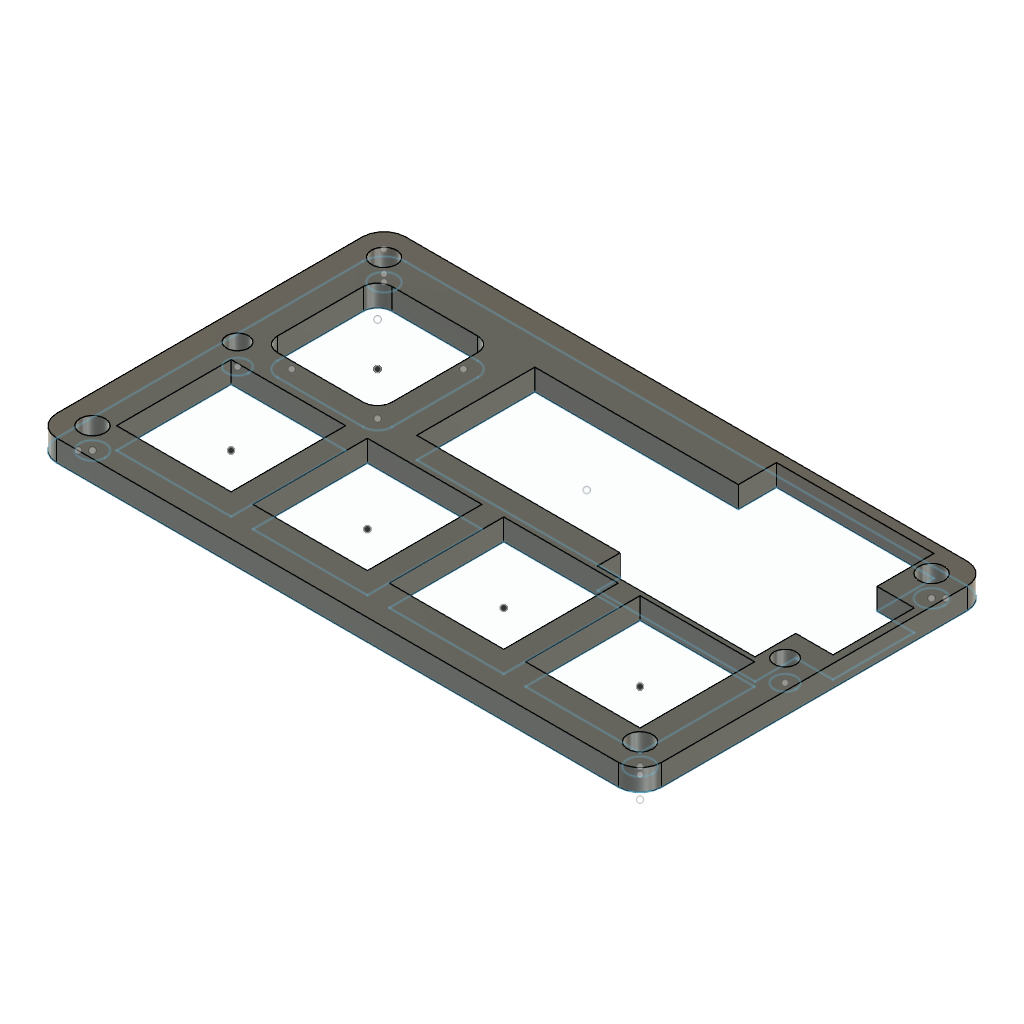
Hayai Upper midplate (Autodesk Fusion 360 design; units mm, degrees)
part number: 2026-09-20-16-56-58-125
Autodesk Fusion 360 part; units mm, degrees
sketch "Sketch1" plane through (0, 0, 0) normal (0, 0, 1) x (1, 0, 0)
  circle A0 centre (-38.26, 20.3675) radius 1.75
  circle A1 centre (38.26, 20.3675) radius 1.75
  circle A2 centre (38.26, -20.3675) radius 1.75
  circle A3 centre (-38.26, -20.3675) radius 1.75
  line L0 (14, 22.9575) -> (36, 22.9575)
  line L1 (36, 15) -> (36, 22.9575)
  line L2 (36, 15) -> (41.21, 15)
  line L3 (41.21, 15) -> (41.21, 3.65)
  line L4 (41.21, 3.65) -> (36, 3.65)
  line L5 (36, -2.0425) -> (36, 3.65)
  line L6 (36, -2.0425) -> (14, -2.0425)
  line L7 (-14.435, 1.1275) -> (-14.435, 17.6275)
  line L8 (-14.435, 1.1275) -> (14, 1.1275)
  line L9 (-14.435, 17.6275) -> (14, 17.6275)
  line L10 (14, -2.0425) -> (14, 1.1275)
  line L11 (14, 17.6275) -> (14, 22.9575)
  circle A4 centre (-38.26, -0.0995) radius 1.525
  circle A5 centre (38.26, -0.0995) radius 1.525
  line L12 (-39.26, 24.3675) -> (39.26, 24.3675)
  line L13 (42.26, 21.3675) -> (42.26, -21.3675)
  line L14 (39.26, -24.3675) -> (-39.26, -24.3675)
  line L15 (-42.26, -21.3675) -> (-42.26, 21.3675)
  arc A6 (-39.26, 24.3675) -> (-42.26, 21.3675) centre (-39.26, 21.3675) ccw
  arc A7 (42.26, 21.3675) -> (39.26, 24.3675) centre (39.26, 21.3675) ccw
  arc A8 (39.26, -24.3675) -> (42.26, -21.3675) centre (39.26, -21.3675) ccw
  arc A9 (-42.26, -21.3675) -> (-39.26, -24.3675) centre (-39.26, -21.3675) ccw
  line L16 (-22.19, 1.4035) -> (-34.19, 1.4035)
  line L17 (-36.19, 3.4035) -> (-36.19, 15.4035)
  line L18 (-34.19, 17.4035) -> (-22.19, 17.4035)
  line L19 (-20.19, 15.4035) -> (-20.19, 3.4035)
  arc A10 (-34.19, 17.4035) -> (-36.19, 15.4035) centre (-34.19, 15.4035) ccw
  arc A11 (-22.19, 1.4035) -> (-20.19, 3.4035) centre (-22.19, 3.4035) ccw
  arc A12 (-36.19, 3.4035) -> (-34.19, 1.4035) centre (-34.19, 3.4035) ccw
  arc A13 (-20.19, 15.4035) -> (-22.19, 17.4035) centre (-22.19, 15.4035) ccw
  line L20 (20.575, -18.6825) -> (36.575, -18.6825)
  line L21 (36.575, -18.6825) -> (36.575, -2.6825)
  line L22 (36.575, -2.6825) -> (20.575, -2.6825)
  line L23 (20.575, -2.6825) -> (20.575, -18.6825)
  line L24 (1.525, -18.6825) -> (17.525, -18.6825)
  line L25 (17.525, -18.6825) -> (17.525, -2.6825)
  line L26 (17.525, -2.6825) -> (1.525, -2.6825)
  line L27 (1.525, -2.6825) -> (1.525, -18.6825)
  line L28 (-17.525, -18.6825) -> (-1.525, -18.6825)
  line L29 (-1.525, -18.6825) -> (-1.525, -2.6825)
  line L30 (-1.525, -2.6825) -> (-17.525, -2.6825)
  line L31 (-17.525, -2.6825) -> (-17.525, -18.6825)
  line L32 (-36.575, -18.6825) -> (-20.575, -18.6825)
  line L33 (-20.575, -18.6825) -> (-20.575, -2.6825)
  line L34 (-20.575, -2.6825) -> (-36.575, -2.6825)
  line L35 (-36.575, -2.6825) -> (-36.575, -18.6825)
  point P0 (1.0651, 9.3775)
  point P1 (-28.19, 9.4035)
  point P2 (-28.19, 9.4035)
  point P3 (42.26, -24.3675)
  point P4 (-42.26, 24.3675)
  point P5 (-28.19, 9.4035)
  point P6 (-28.19, 9.4035)
  point P7 (28.575, -10.6825)
  point P8 (9.525, -10.6825)
  point P9 (-28.575, -10.6825)
  point P10 (-9.525, -10.6825)
  point P11 (28.575, -10.6825)
  point P12 (9.525, -10.6825)
  point P13 (-9.525, -10.6825)
  point P14 (-28.575, -10.6825)
  dimension "d2" = 3.5
  dimension "d11" = 22
  dimension "d12" = 25
  dimension "d13" = 5.21
  dimension "d14" = 11.35
  dimension "d18" = 16.5
  dimension "d31" = 3.05
  dimension "d32" = 3.05
  dimension "d33" = 20.268
  dimension "d34" = 20.268
  dimension "d53" = 3
  dimension "d54" = 3
  dimension "d55" = 3
  dimension "d56" = 3
  dimension "d67" = 84.52
  dimension "d68" = 14.07
  dimension "d69" = 14.964
  dimension "d72" = 2
  dimension "d73" = 2
  dimension "d74" = 2
  dimension "d75" = 2
  dimension "d80" = 19.05
  dimension "d81" = 16
  dimension "d82" = 16
  dimension "d83" = 16
  dimension "d84" = 16
  dimension "d85" = 16
  dimension "d86" = 16
  dimension "d87" = 16
  dimension "d88" = 16
  constraint horizontal L0
  constraint horizontal L6
  constraint horizontal L2
  constraint vertical L3
  constraint horizontal L4
  constraint perpendicular L8 L10
  constraint coincident P6 P5
  constraint horizontal L12
  constraint vertical L13
  constraint horizontal L14
  constraint vertical L15
  constraint tangent L12 A6
  constraint tangent L15 A6
  constraint tangent L12 A7
  constraint tangent L13 A7
  constraint tangent L13 A8
  constraint tangent L14 A8
  constraint tangent L14 A9
  constraint tangent L15 A9
  constraint horizontal L16
  constraint perpendicular L16 L17
  constraint parallel L16 L18
  constraint parallel L17 L19
  constraint tangent L18 A10
  constraint tangent L17 A10
  constraint tangent L16 A11
  constraint tangent L19 A11
  constraint tangent L16 A12
  constraint tangent L17 A12
  constraint tangent L18 A13
  constraint tangent L19 A13
  constraint horizontal L20
  constraint perpendicular L20 L21
  constraint parallel L20 L22
  constraint parallel L21 L23
  constraint coincident P11 P7
  constraint horizontal L24
  constraint perpendicular L24 L25
  constraint parallel L24 L26
  constraint parallel L25 L27
  constraint coincident P12 P8
  constraint horizontal L28
  constraint perpendicular L28 L29
  constraint parallel L28 L30
  constraint parallel L29 L31
  constraint coincident P13 P10
  constraint horizontal L32
  constraint perpendicular L32 L33
  constraint parallel L32 L34
  constraint parallel L33 L35
  constraint coincident P14 P9
  constraint equal A0 A3
  constraint equal A0 A2
  constraint equal A0 A1
  measures "d2" diameter of A0
  measures "d11" distance of L0.end L0.start
  measures "d12" distance of L6.end L0.start
  measures "d13" distance of L1.start L2.end
  measures "d14" distance of L1.start L4.end
  measures "d18" distance of L7.start L7.end
  measures "d31" diameter of A4
  measures "d32" diameter of A5
  measures "d33" distance of A2.centre A5.centre
  measures "d34" distance of A3.centre A4.centre
  measures "d53" radius of A6
  measures "d54" radius of A7
  measures "d55" radius of A8
  measures "d56" radius of A9
  measures "d67" distance of L13 L15
  measures "d68" distance of L15 P6
  measures "d69" distance of L12 P6
  measures "d72" radius of A10
  measures "d73" radius of A11
  measures "d74" radius of A12
  measures "d75" radius of A13
  measures "d80" distance of P14 P13
  measures "d81" distance of L21.end L22.end
  measures "d82" distance of L20.end L21.end
  measures "d83" distance of L25.end L26.end
  measures "d84" distance of L24.end L25.end
  measures "d85" distance of L29.end L30.end
  measures "d86" distance of L28.end L29.end
  measures "d87" distance of L33.end L34.end
  measures "d88" distance of L32.end L33.end
extrude "Extrude13" add sketch "Sketch1" along normal blind 3 contours L12 L13 L14 L15 A6 A7 A8 A9 | L16 L17 L18 L19 A10 A11 A12 A13 | L20 L21 L22 L23 | L24 L25 L26 L27 | L28 L29 L30 L31 | L32 L33 L34 L35 makes body 1
extrude "Extrude14" add sketch "Sketch1" along normal blind 3 separate body contours L12 L13 L14 L15 A6 A7 A8 A9 | L20 L21 L22 L23 | L24 L25 L26 L27 | L28 L29 L30 L31 | L32 L33 L34 L35 makes body 2
extrude "Extrude15" cut sketch "Sketch1" along normal blind 3 contours L16 L17 L18 L19 A10 A11 A12 A13 bodies 1
extrude "Extrude16" add sketch "Sketch1" along normal blind 3 separate body makes body 3
extrude "Extrude17" cut sketch "Sketch1" along normal blind 3 contours L20 L21 L22 L23 | L24 L25 L26 L27 | L28 L29 L30 L31 | L32 L33 L34 L35 bodies 1 2
extrude "Extrude18" add sketch "Sketch1" along normal blind 3 separate body makes body 4
